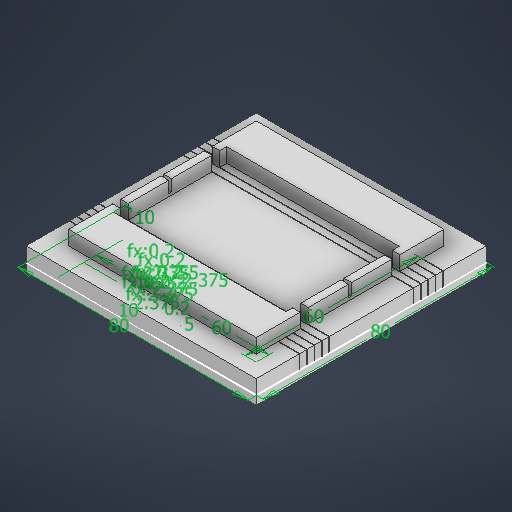
# Autodesk Inventor part: Cortador Ancho PDMS4
Saved by Autodesk Inventor 2026.1 (Build 301233000, 233)
## iProperties
Created: 2025-10-29
Part Number: Cortador Ancho PDMS4
Material: Genérico
Document SubType Name: Modeling
Designer: Laboratorio_sensores
Density: 1 g/cm^3
Appearance: Valor por defecto
Author: Laboratorio_sensores
Autodesk Inventor part; units mm, degrees
ref_plane "YZ Plane" through (0, 0, 0) normal (1, 0, 0) x (0, 1, 0)
ref_plane "XZ Plane" through (0, 0, 0) normal (0, 1, 0) x (-1, 0, 0)
ref_plane "XY Plane" through (0, 0, 0) normal (0, 0, 1) x (1, 0, 0)
sketch "Boceto1" plane through (0, 0, 0) normal (0, 1, 0) x (-1, 0, 0)
  line L0 (0, 0) -> (80, 0)
  line L1 (80, 0) -> (80, -80)
  line L2 (80, -80) -> (0, -80)
  line L3 (0, -80) -> (0, 0)
  line L4 (10, -70) -> (70, -70)
  line L5 (70, -70) -> (70, -10)
  line L6 (70, -10) -> (10, -10)
  line L7 (10, -10) -> (10, -70)
  line L8 (0, -12.375) -> (80, -12.375)
  line L9 (0, -14.95) -> (80, -14.95)
  line L10 (0, -17.525) -> (80, -17.525)
  line L11 (80, -20.1) -> (0, -20.1)
  line L12 (0, -22.675) -> (80, -22.675)
  line L13 (0, -12.575) -> (80, -12.575)
  line L14 (0, -15.15) -> (80, -15.15)
  line L15 (0, -17.725) -> (80, -17.725)
  line L16 (80, -20.3) -> (0, -20.3)
  line L17 (0, -22.875) -> (80, -22.875)
  line L18 (0, -25.25) -> (80, -25.25)
  line L19 (0, -25.45) -> (80, -25.45)
  line L20 (10, -40) -> (80, -40)
  line L21 (0, -67.625) -> (80, -67.625)
  line L22 (0, -65.05) -> (80, -65.05)
  line L23 (0, -62.475) -> (80, -62.475)
  line L24 (80, -59.9) -> (0, -59.9)
  line L25 (0, -57.325) -> (80, -57.325)
  line L26 (0, -67.425) -> (80, -67.425)
  line L27 (0, -64.85) -> (80, -64.85)
  line L28 (0, -62.275) -> (80, -62.275)
  line L29 (80, -59.7) -> (0, -59.7)
  line L30 (0, -57.125) -> (80, -57.125)
  line L31 (0, -54.75) -> (80, -54.75)
  line L32 (0, -54.55) -> (80, -54.55)
  line L33 (72.625, -7.375) -> (7.375, -7.375)
  line L34 (7.375, -7.375) -> (7.375, -72.625)
  line L35 (7.375, -72.625) -> (72.625, -72.625)
  line L36 (72.625, -72.625) -> (72.625, -7.375)
  line L37 (7.375, 0) -> (0, 0)
  line L38 (7.375, -80) -> (0, -80)
  point P0 (10, -12.375)
  point P1 (70, -12.375)
  point P2 (10, -14.95)
  point P3 (70, -14.95)
  point P4 (10, -17.525)
  point P5 (70, -17.525)
  point P6 (70, -20.1)
  point P7 (10, -20.1)
  point P8 (10, -22.675)
  point P9 (70, -22.675)
  point P10 (10, -12.575)
  point P11 (70, -12.575)
  point P12 (10, -15.15)
  point P13 (70, -15.15)
  point P14 (10, -17.725)
  point P15 (70, -17.725)
  point P16 (70, -20.3)
  point P17 (10, -20.3)
  point P18 (10, -22.875)
  point P19 (70, -22.875)
  point P20 (10, -25.25)
  point P21 (70, -25.25)
  point P22 (10, -25.45)
  point P23 (70, -25.45)
  point P24 (10, -67.625)
  point P25 (70, -67.625)
  point P26 (10, -65.05)
  point P27 (70, -65.05)
  point P28 (10, -62.475)
  point P29 (70, -62.475)
  point P30 (70, -59.9)
  point P31 (10, -59.9)
  point P32 (10, -57.325)
  point P33 (70, -57.325)
  point P34 (10, -67.425)
  point P35 (70, -67.425)
  point P36 (10, -64.85)
  point P37 (70, -64.85)
  point P38 (10, -62.275)
  point P39 (70, -62.275)
  point P40 (70, -59.7)
  point P41 (10, -59.7)
  point P42 (10, -57.125)
  point P43 (70, -57.125)
  point P44 (10, -54.75)
  point P45 (70, -54.75)
  point P46 (10, -54.55)
  point P47 (70, -54.55)
  point P48 (72.625, -12.375)
  point P49 (7.375, -12.375)
  point P50 (72.625, -54.55)
  point P51 (72.625, -25.45)
  point P52 (70, -25.45)
  point P53 (70, -54.55)
  point P54 (7.375, -25.45)
  point P55 (7.375, -54.55)
  point P56 (10, -54.55)
  point P57 (10, -25.45)
  point P58 (10, -67.625)
  point P59 (7.375, -67.625)
  point P60 (72.625, -67.625)
  point P61 (70, -67.625)
  point P62 (7.375, -14.95)
  point P63 (72.625, -14.95)
  point P64 (72.625, -65.05)
  point P65 (70, -65.05)
  point P66 (10, -65.05)
  point P67 (7.375, -65.05)
  point P68 (70, -67.425)
  point P69 (10, -67.425)
  point P70 (10, -12.575)
  point P71 (70, -12.575)
  point P72 (72.625, -64.85)
  point P73 (7.375, -64.85)
  point P74 (7.375, -15.15)
  point P75 (70, -15.15)
  point P76 (7.375, -62.475)
  point P77 (10, -64.85)
  point P78 (10, -62.475)
  point P79 (72.625, -62.475)
  point P80 (70, -62.475)
  point P81 (70, -64.85)
  point P82 (7.375, -17.525)
  point P83 (10, -15.15)
  point P84 (72.625, -17.525)
  point P85 (72.625, -20.1)
  point P86 (7.375, -20.1)
  point P87 (72.625, -59.9)
  point P88 (70, -59.9)
  point P89 (70, -62.275)
  point P90 (10, -62.275)
  point P91 (10, -59.9)
  point P92 (7.375, -59.9)
  point P93 (10, -17.725)
  point P94 (70, -17.725)
  point P95 (72.625, -57.325)
  point P96 (70, -57.325)
  point P97 (70, -59.7)
  point P98 (10, -59.7)
  point P99 (10, -57.325)
  point P100 (7.375, -57.325)
  point P101 (7.375, -22.675)
  point P102 (10, -20.3)
  point P103 (70, -20.3)
  point P104 (72.625, -22.675)
  dimension "d5" = 10
  dimension "d0" = 80
  dimension "d1" = 80
  dimension "d2" = 60
  dimension "d3" = 60
  dimension "d4" = 10
  dimension "d6" = 2.375
  dimension "d7" = 0.2
  dimension "d8" = 2.375
  dimension "d9" = 0.2
  dimension "d10" = 0.2
  dimension "d11" = 0.2
  dimension "d12" = 0.2
  dimension "d13" = 2.375
  dimension "d14" = 2.375
  dimension "d15" = 2.375
  dimension "d16" = 2.375
  dimension "d17" = 0.2
  dimension "d35" = 5
  constraints: 70 end point, 50 point on line, 24 symmetric about line, 11 parallel, 9 horizontal, 3 perpendicular, 75 other
  measures "d0" distance of L0.start L0.end
  measures "d1" distance of L2.end L0.start
  measures "d2" distance of L6.end L4.start
  measures "d3" distance of L6.start L6.end
  measures "d4" distance between parallel lines of L0 L6
  measures "d6" distance between parallel lines of L6 L8
  measures "d7" distance between parallel lines of L8 L13
  measures "d8" distance between parallel lines of L9 L13
  measures "d9" distance between parallel lines of L9 L14
  measures "d10" distance between parallel lines of L15 L10
  measures "d11" distance between parallel lines of L16 L11
  measures "d12" distance between parallel lines of L17 L12
  measures "d13" distance between parallel lines of L10 L14
  measures "d14" distance between parallel lines of L11 L15
  measures "d15" distance between parallel lines of L16 L12
  measures "d16" distance between parallel lines of L18 L17
  measures "d17" distance between parallel lines of L18 L19
  measures "d35" distance between parallel lines of L33 L8
extrude "Extrusión1" add sketch "Boceto1" along normal blind 5 contours L0 L1 L8 L36 L33 L34 L3 | L8 L34 L13 L3 | L13 L34 L9 L3 | L34 L33 L36 L8 L5 L6 L7 | L8 L7 L13 L34 | L1 L13 L36 L8 | L13 L7 L9 L34 | L8 L5 L13 L7 | L7 L6 L5 L8 | L1 L9 L36 L13 | L36 L13 L5 L8 | L14 L34 L10 L3 | L13 L5 L9 L7 | L36 L9 L5 L13 | L14 L7 L10 L34 | L1 L10 L36 L14 | L15 L34 L11 L3 | L14 L5 L10 L7 | L36 L10 L5 L14 | L15 L7 L11 L34 | L1 L11 L36 L15 | L16 L34 L12 L3 | L15 L5 L11 L7 | L36 L11 L5 L15 | L16 L7 L12 L34 | L1 L12 L36 L16 | L17 L34 L18 L3 | L16 L5 L12 L7 | L36 L12 L5 L16 | L17 L7 L18 L34 | L1 L18 L36 L17 | L19 L34 L32 L3 | L17 L5 L18 L7 | L36 L18 L5 L17 | L19 L7 L32 L34 | L1 L20 L36 L19 | L31 L34 L30 L3 | L19 L5 L20 L7 | L1 L32 L36 L20 | L36 L20 L5 L19 | L31 L7 L30 L34 | L7 L20 L5 L32 | L36 L32 L5 L20 | L25 L34 L29 L3 | L31 L5 L30 L7 | L1 L30 L36 L31 | L25 L7 L29 L34 | L31 L36 L30 L5 | L24 L34 L28 L3 | L25 L5 L29 L7 | L1 L29 L36 L25 | L24 L7 L28 L34 | L25 L36 L29 L5 | L23 L34 L27 L3 | L24 L5 L28 L7 | L1 L28 L36 L24 | L23 L7 L27 L34 | L24 L36 L28 L5 | L22 L34 L26 L3 | L23 L5 L27 L7 | L1 L27 L36 L23 | L26 L34 L21 L3 | L22 L7 L26 L34 | L23 L36 L27 L5 | L21 L34 L35 L36 L1 L2 L3 | L26 L7 L21 L34 | L22 L5 L26 L7 | L1 L26 L36 L22 | L21 L7 L4 L5 L36 L35 L34 | L26 L5 L21 L7 | L22 L36 L26 L5 | L1 L21 L36 L26 | L21 L5 L4 L7 | L26 L36 L21 L5
sketch "Boceto2" plane through (0, 0, 0) normal (0, -1, 0) x (1, 0, 0)
  line L0 (0, -80) -> (-80, -80) projected
  line L1 (-80, 0) -> (0, 0) projected
  line L2 (-80, -80) -> (-80, 0)
  line L3 (-80, 0) -> (0, 0)
  line L4 (-80, -65.05) -> (0, -65.05) construction
  line L5 (0, 0) -> (0, -80)
  line L6 (-80, -80) -> (0, -80)
  constraints: 8 end point, 2 perpendicular, 1 parallel, 1 vertical
extrude "Extrusión4" add sketch "Boceto2" along normal blind 3
extrude "Extrusión5" add sketch "Boceto1" along normal blind 10 contours L34 L33 L36 L8 L5 L6 L7 | L8 L7 L13 L34 | L13 L7 L9 L34 | L8 L5 L13 L7 | L7 L6 L5 L8 | L36 L13 L5 L8 | L9 L7 L14 L34 | L13 L5 L9 L7 | L36 L9 L5 L13 | L14 L7 L10 L34 | L9 L5 L14 L7 | L36 L14 L5 L9 | L10 L7 L15 L34 | L14 L5 L10 L7 | L36 L10 L5 L14 | L15 L7 L11 L34 | L10 L5 L15 L7 | L36 L15 L5 L10 | L11 L7 L16 L34 | L15 L5 L11 L7 | L36 L11 L5 L15 | L16 L7 L12 L34 | L11 L5 L16 L7 | L36 L16 L5 L11 | L36 L12 L5 L16 | L19 L7 L32 L34 | L36 L20 L5 L19 | L36 L32 L5 L20 | L25 L7 L29 L34 | L29 L7 L24 L34 | L24 L7 L28 L34 | L29 L5 L24 L7 | L25 L36 L29 L5 | L28 L7 L23 L34 | L24 L5 L28 L7 | L29 L36 L24 L5 | L23 L7 L27 L34 | L28 L5 L23 L7 | L24 L36 L28 L5 | L27 L7 L22 L34 | L23 L5 L27 L7 | L28 L36 L23 L5 | L22 L7 L26 L34 | L27 L5 L22 L7 | L23 L36 L27 L5 | L26 L7 L21 L34 | L22 L5 L26 L7 | L27 L36 L22 L5 | L21 L7 L4 L5 L36 L35 L34 | L26 L5 L21 L7 | L22 L36 L26 L5 | L21 L5 L4 L7 | L26 L36 L21 L5
sketch "Boceto3" plane through (0, 10, 0) normal (0, 1, 0) x (1, 0, 0)
  line L0 (-7.375, 25.45) -> (-7.375, 54.55) projected
  line L1 (-7.375, 40) -> (-86.5517, 40)
  line L2 (-5, 39.5) -> (-84.1767, 39.5)
  line L3 (-5, 40.5) -> (-84.1767, 40.5)
  line L4 (-10, 54.55) -> (-10, 25.45) projected
  line L5 (-5, 40.5) -> (-5, 39.5)
  line L6 (-84.1767, 40.5) -> (-84.1767, 39.5)
  point P0 (0, 0)
  point P1 (-10, 40)
  point P2 (-10, 39.5)
  point P3 (-10, 40.5)
  point P4 (-7.375, 39.5)
  point P5 (-7.375, 40.5)
  dimension "d31" = 0.5
  dimension "d32" = 0.5
  constraints: 10 end point, 3 parallel, 2 midpoint, 1 horizontal, 1 perpendicular
  measures "d31" distance from line of point (-10, 40) L2
  measures "d32" distance between parallel lines of L1 L3
extrude "Extrusión6" cut sketch "Boceto3" against normal blind 4 contours L2 L4 L1 L0 | L1 L4 L3 L0 | L2 L6 L1 L4 | L1 L6 L3 L4
equation "\"d8\" = d6"
equation "\"d9\" = d7"
equation "\"d10\" = d9"
equation "\"d11\" = d7"
equation "\"d12\" = d7"
equation "\"d13\" = d6"
equation "\"d14\" = d6"
equation "\"d15\" = d6"
equation "\"d16\" = d6"
equation "\"d17\" = d7"
